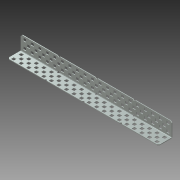
# Autodesk Inventor part: Bumper 20 Hole
Saved by Autodesk Inventor 2013 (Build 170138000, 138)
## iProperties
Category: Structure
Company: Autodesk Inc.
Created: 2012-03-22
Part Number: Bumper 20 Hole
Material: Steel
Document SubType Name: Sheet Metal
Designer: Autodesk Inc.
Density: 7.85 g/cm^3
Sheet Metal Rule: Default
Vendor: VEX
Author: Autodesk Inc.
Autodesk Inventor part; units mm, degrees
ref_plane "YZ Plane" through (0, 0, 0) normal (1, 0, 0) x (0, 1, 0)
ref_plane "XZ Plane" through (0, 0, 0) normal (0, 1, 0) x (-1, 0, 0)
sketch "Sketch1" plane through (0, 0, 0) normal (0, 0, 1) x (1, 0, 0)
  line L0 (0.7045, -0.4445) -> (254.7045, -0.4445)
  line L1 (254.7045, -0.4445) -> (254.7045, 22.9743)
  line L2 (254.7045, 22.9743) -> (0.7045, 22.9743)
  line L3 (0.7045, 22.9743) -> (0.7045, -0.4445)
  point P0 (0, 0)
  dimension "d0" = 254
  dimension "d1" = 23.4188
  measures "d0" distance of L2.end L1.end
  measures "d1" distance of L0.end L1.end
extrude "Plate1" add sketch "Sketch1" along normal blind 1.17
sketch "Sketch2" plane through (0.7045, 21.8043, 0) normal (0, 1, 0) x (-1, 0, 0)
  line L0 (-254, 0) -> (0, 0)
  line L1 (0, 0) -> (0, 24.5888)
  line L2 (0, 24.5888) -> (-254, 24.5888)
  line L3 (-254, 24.5888) -> (-254, 0)
  constraints: 6 end point, 1 horizontal, 1 perpendicular, 1 vertical
edge flange "Flange1" height 23.4188 angle 90 thickness 1.17 bend radius 0.8139 thickness toward (0, 1, 0) relief tear relief width 1.17 relief depth 0.585 edges at (127.7045, 22.9743, 1.17) wall of the first edge with corners at (254.7045, 21.8043, 0) (0.7045, 21.8043, 0) (0.7045, 21.8043, 24.5888) (254.7045, 21.8043, 24.5888)
bend "Bend1"
corner "Corner1"
sketch "Sketch3" plane through (254.7045, 21.8043, 24.5888) normal (1, 0, 0) x (0, 0, -1)
  line L0 (22.6049, 0) -> (22.6049, 1.17) projected
  line L1 (22.6049, 1.17) -> (0, 1.17) projected
  line L2 (0, 0) -> (0, 1.17) projected
  line L3 (0, 0) -> (22.6049, 0) projected
  line L4 (22.6049, 0) -> (22.6049, 1.17) projected
  arc A0 (23.4188, -0.8139) -> (22.6049, 0) centre (22.6049, -0.8139) ccw projected
  line L5 (24.5888, -0.8139) -> (23.4188, -0.8139) projected
  arc A1 (24.5888, -0.8139) -> (22.6049, 1.17) centre (22.6049, -0.8139) ccw projected
  line L6 (24.5888, -0.8139) -> (23.4188, -0.8139) projected
  line L7 (23.4188, -0.8139) -> (23.4188, -22.2488) projected
  line L8 (24.5888, -22.2488) -> (23.4188, -22.2488) projected
  line L9 (24.5888, -22.2488) -> (24.5888, -0.8139) projected
  point P0 (24.5888, -21.8043)
  dimension "d13" = 0.8139
  dimension "d14" = 1.9839
  measures "d13" radius of A0
  measures "d14" radius of A1
sketch "Sketch4" plane through (0.7045, 22.9743, 24.5888) normal (0, 1, 0) x (1, 0, 0)
  line L0 (254, 0) -> (0, 0) projected
  line L1 (254, 22.6049) -> (254, 0) projected
  line L2 (249.4534, 2.8702) -> (245.8466, 2.8702)
  line L3 (245.3386, 3.3782) -> (245.3386, 6.985)
  line L4 (245.8466, 7.493) -> (249.4534, 7.493)
  line L5 (249.9614, 6.985) -> (249.9614, 3.3782)
  arc A0 (249.4534, 2.8702) -> (249.9614, 3.3782) centre (249.4534, 3.3782) ccw
  arc A1 (245.3386, 3.3782) -> (245.8466, 2.8702) centre (245.8466, 3.3782) ccw
  arc A2 (245.8466, 7.493) -> (245.3386, 6.985) centre (245.8466, 6.985) ccw
  arc A3 (249.9614, 6.985) -> (249.4534, 7.493) centre (249.4534, 6.985) ccw
  point P0 (-0.7045, 24.5888)
  point P1 (249.9614, 2.8702)
  point P2 (245.3386, 7.493)
  point P3 (245.3386, 2.8702)
  dimension "d15" = 4.6228
  dimension "d16" = 4.6228
  dimension "d17" = 2.8702
  dimension "d18" = 4.0386
  dimension "d19" = 0.508
  constraints: 8 end point, 8 point on circle, 8 tangent, 6 point on line, 4 centre point, 3 equal radius, 2 parallel, 1 horizontal, 1 perpendicular
  measures "d15" distance of point (249.961, 2.87) point (245.339, 2.87)
  measures "d16" distance of point (245.339, 2.87) point (245.339, 7.493)
  measures "d17" distance between parallel lines of L0 L2
  measures "d18" distance between parallel lines of L5 L1
  measures "d19" radius of A0
extrude "Cut1" cut sketch "Sketch4" against normal blind 1.17
pattern_linear "Rectangular Pattern1" count 20 spacing 12.7 along (-1, 0, 0) count 2 spacing 12.7 along (0, 0, -1) of "Cut1"
sketch "Sketch5" plane through (0.7045, 22.9743, 24.5888) normal (0, 1, 0) x (1, 0, 0)
  line L0 (249.4534, 2.8702) -> (245.8466, 2.8702) projected
  line L1 (249.9614, 6.985) -> (249.9614, 3.3782) projected
  line L2 (243.1034, 9.2202) -> (239.4966, 9.2202)
  line L3 (238.9886, 9.7282) -> (238.9886, 13.335)
  line L4 (239.4966, 13.843) -> (243.1034, 13.843)
  line L5 (243.6114, 13.335) -> (243.6114, 9.7282)
  arc A0 (243.1034, 9.2202) -> (243.6114, 9.7282) centre (243.1034, 9.7282) ccw
  arc A1 (238.9886, 9.7282) -> (239.4966, 9.2202) centre (239.4966, 9.7282) ccw
  arc A2 (239.4966, 13.843) -> (238.9886, 13.335) centre (239.4966, 13.335) ccw
  arc A3 (243.6114, 13.335) -> (243.1034, 13.843) centre (243.1034, 13.335) ccw
  point P0 (-0.7045, 24.5888)
  point P1 (243.6114, 9.2202)
  point P2 (238.9886, 13.843)
  point P3 (238.9886, 9.2202)
  point P4 (243.6114, 13.843)
  dimension "d28" = 4.6228
  dimension "d29" = 4.6228
  dimension "d30" = 6.35
  dimension "d31" = 6.35
  dimension "d34" = 0.508
  constraints: 8 end point, 8 point on circle, 8 point on line, 8 tangent, 4 centre point, 3 equal radius, 2 parallel, 1 horizontal, 1 perpendicular
  measures "d28" distance of point (243.611, 9.22) point (238.989, 9.22)
  measures "d29" distance of point (238.989, 9.22) point (238.989, 13.843)
  measures "d30" distance between parallel lines of L5 L1
  measures "d31" distance between parallel lines of L2 L0
  measures "d34" radius of A0
extrude "Cut2" cut sketch "Sketch5" against normal blind 1.17
pattern_linear "Rectangular Pattern2" count 19 spacing 12.7 along (-1, 0, 0) of "Cut2"
sketch "Sketch6" plane through (0.7045, 22.9743, 24.5888) normal (0, 1, 0) x (1, 0, 0)
  circle A0 centre (6.35, 17.8816) radius 2.3114
  line L0 (4.5466, 20.193) -> (8.1534, 20.193) projected
  line L1 (8.6614, 19.685) -> (8.6614, 16.0782) projected
  point P0 (-0.7045, 24.5888)
  constraints: 2 tangent, 1 centre point
surface extrude "ExtrusionSrf1" sketch "Sketch6" against normal up to surface (1.17 mm away) shown no curves A0
pattern_linear "Rectangular Pattern3" count 20 spacing 12.7 along (1, 0, 0) count 2 spacing 12.7 along (0, 0, 1) of "ExtrusionSrf1"
sketch "Sketch7" plane through (0.7045, 22.9743, 24.5888) normal (0, 1, 0) x (1, 0, 0)
  line L0 (10.8966, 13.843) -> (14.5034, 13.843) projected
  line L1 (15.0114, 13.335) -> (15.0114, 9.7282) projected
  circle A0 centre (12.7, 11.5316) radius 2.3114
  point P0 (-0.7045, 24.5888)
  constraints: 2 tangent, 1 centre point
surface extrude "ExtrusionSrf401" sketch "Sketch7" against normal up to surface (1.17 mm away) shown no curves A0
pattern_linear "Rectangular Pattern4" count 19 spacing 12.7 along (1, 0, 0) of "ExtrusionSrf401"
ref_plane "Work Plane1" through (127.7045, 20.9904, 1.9839) normal (0, 0.7071068, 0.7071068) x (1, 0, 0)
mirror "Mirror1" about plane through (127.7045, 20.9904, 1.9839) normal (0, 0.7071068, 0.7071068) of "Cut1", "Rectangular Pattern1", "Cut2", "Rectangular Pattern2", "ExtrusionSrf1", "Rectangular Pattern3", "ExtrusionSrf401", "Rectangular Pattern4"
chamfer "Corner Chamfer1" distance 2.286 angle 45 4 edges at (0.7045, 22.3893, 24.5888) (254.7045, -0.4445, 0.585) (254.7045, 22.3893, 24.5888) (0.7045, -0.4445, 0.585)
sketch "Sketch8" plane through (0.7045, 22.9743, 1.9839) normal (0, 1, 0) x (1, 0, 0)
  line L0 (251.714, -22.6049) -> (2.286, -22.6049) projected
  line L1 (254, -20.3189) -> (251.714, -22.6049) projected
  line L2 (65.3034, -13.3847) -> (61.6966, -13.3847) projected
  line L3 (61.468, -22.6049) -> (63.5, -20.5729)
  line L4 (63.5, -20.5729) -> (65.532, -22.6049)
  point P0 (-0.7045, 1.9839)
  point P1 (63.5, -13.3847)
  dimension "d173" = 4.064
  constraints: 4 end point, 2 point on line, 1 midpoint, 1 parallel, 1 perpendicular, 1 vertical alignment
  measures "d173" distance of L4.end L3.start
extrude "Cut3" cut sketch "Sketch8" against normal blind 1.17
pattern_linear "Rectangular Pattern5" count 3 spacing 63.5 along (1, 0, 0) of "Cut3"
sketch "Sketch9" plane through (0, 0, 0) normal (0, 0, -1) x (-1, 0, 0)
  line L0 (-189.4011, 7.6057) -> (-193.0079, 7.6057) projected
  line L1 (-252.4185, -0.4445) -> (-254.7045, 1.8415) projected
  line L2 (-2.9905, -0.4445) -> (-252.4185, -0.4445) projected
  line L3 (-193.2365, -0.4445) -> (-191.2045, 1.5875)
  line L4 (-191.2045, 1.5875) -> (-189.1725, -0.4445)
  point P0 (0, 0)
  point P1 (-191.2045, 7.6057)
  dimension "d179" = 4.064
  constraints: 4 end point, 2 point on line, 1 midpoint, 1 parallel, 1 perpendicular, 1 vertical alignment
  measures "d179" distance of L4.end L3.start
extrude "Cut4" cut sketch "Sketch9" against normal blind 1.17
pattern_linear "Rectangular Pattern6" count 3 spacing 63.5 along (-1, 0, 0) of "Cut4"
sketch "Sketch10" plane through (0.7045, 22.9743, 1.9839) normal (0, 1, 0) x (1, 0, 0)
  line L0 (61.6966, -8.7619) -> (65.3034, -8.7619) projected
  line L1 (254, 0) -> (0, 0) projected
  line L2 (0, 1.9839) -> (254, 1.9839) projected
  line L3 (61.1543, 0.992) -> (65.8457, 0.992) construction
  line L4 (61.1543, 0.992) -> (63.5, -1.1684)
  line L5 (63.5, -1.1684) -> (65.8457, 0.992)
  line L6 (61.1543, 0.992) -> (63.5, 3.1523)
  line L7 (65.8457, 0.992) -> (63.5, 3.1523)
  point P0 (-0.7045, 1.9839)
  point P1 (63.5, -8.7619)
  point P2 (63.5, 0.992)
  point P3 (63.5, -8.7619)
  dimension "d186" = 1.9839
  dimension "d190" = 0.992
  dimension "d191" = 94.71
  dimension "d192" = 1.1684
  constraints: 10 end point, 3 midpoint, 3 vertical alignment, 1 equal length, 1 horizontal, 1 parallel
  measures "d186" distance between parallel lines of L2 L1
  measures "d190" distance between parallel lines of L3 L1
  measures "d191" angle of L5 L4
  measures "d192" distance from line of L4.end L1
cut across bends "Cut5" sketch "Sketch10" k factor 0.44
pattern_linear "Rectangular Pattern7" count 3 spacing 63.5 along (1, 0, 0) of "Cut5"
equation "\"d16\" = d15"
equation "\"d20\" = Thickness"
equation "\"d29\" = d28"
equation "\"d31\" = d30"
equation "\"d32\" = Thickness"
equation "\"d3\" = BendReliefWidth"
equation "\"d4\" = BendReliefDepth"
equation "\"d5\" = MinimumRemnant"
equation "\"d6\" = BendRadius"
equation "\"d9\" = BendRadius"
equation "\"d10\" = CornerReliefSize"
equation "\"d11\" = GapSize"
equation "\"d12\" = JacobiRadiusSize"
equation "\"BendReliefWidth\" = Thickness"
equation "\"BendReliefDepth\" = 0.5 * Thickness"
equation "\"CornerReliefSize\" = 4 * Thickness"
equation "\"MinimumRemnant\" = 2 * Thickness"
equation "\"TransitionRadius\" = BendRadius"
equation "\"JacobiRadiusSize\" = BendRadius"
equation "\"GapSize\" = Thickness"
equation "\"d2\" = BendRadius"
equation "\"Thickness\" = 1.17"
equation "\"BendRadius\" = 0.813913"
body "Solid1"
body "Srf1"
body "Srf2"
body "Srf3"
body "Srf4"
body "Srf5"
body "Srf6"
body "Srf7"
body "Srf8"
body "Srf9"
body "Srf10"
body "Srf11"
body "Srf12"
body "Srf13"
body "Srf14"
body "Srf15"
body "Srf16"
body "Srf17"
body "Srf18"
body "Srf19"
body "Srf20"
body "Srf21"
body "Srf22"
body "Srf23"
body "Srf24"
body "Srf25"
body "Srf26"
body "Srf27"
body "Srf28"
body "Srf29"
body "Srf30"
body "Srf31"
body "Srf32"
body "Srf33"
body "Srf34"
body "Srf35"
body "Srf36"
body "Srf37"
body "Srf38"
body "Srf39"
body "Srf40"
body "Srf401"
body "Srf402"
body "Srf403"
body "Srf404"
body "Srf405"
body "Srf406"
body "Srf407"
body "Srf408"
body "Srf409"
body "Srf410"
body "Srf411"
body "Srf412"
body "Srf413"
body "Srf414"
body "Srf415"
body "Srf416"
body "Srf417"
body "Srf418"
body "Srf419"
body "Srf439"
body "Srf440"
body "Srf441"
body "Srf442"
body "Srf443"
body "Srf444"
body "Srf445"
body "Srf446"
body "Srf447"
body "Srf448"
body "Srf449"
body "Srf450"
body "Srf451"
body "Srf452"
body "Srf453"
body "Srf454"
body "Srf455"
body "Srf456"
body "Srf457"
body "Srf458"
body "Srf459"
body "Srf460"
body "Srf461"
body "Srf462"
body "Srf463"
body "Srf464"
body "Srf465"
body "Srf466"
body "Srf467"
body "Srf468"
body "Srf469"
body "Srf470"
body "Srf471"
body "Srf472"
body "Srf473"
body "Srf474"
body "Srf475"
body "Srf476"
body "Srf477"
body "Srf478"
body "Srf420"
body "Srf421"
body "Srf422"
body "Srf423"
body "Srf424"
body "Srf425"
body "Srf426"
body "Srf427"
body "Srf428"
body "Srf429"
body "Srf430"
body "Srf431"
body "Srf432"
body "Srf433"
body "Srf434"
body "Srf435"
body "Srf436"
body "Srf437"
body "Srf438"
